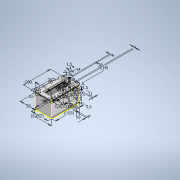
# Autodesk Inventor part: Box-Bildschirm.v2
Saved by Autodesk Inventor 2020 (Build 240168000, 168)
## iProperties
Created: 2019-08-23
Part Number: Box-Bildschirm.v2
Material: Generisch
Document SubType Name: Modeling
Designer: Admin
Density: 1 g/cm^3
Appearance: Vorgabe
Author: Admin
Autodesk Inventor part; units mm, degrees
ref_plane "YZ Plane" through (0, 0, 0) normal (1, 0, 0) x (0, 1, 0)
ref_plane "XZ Plane" through (0, 0, 0) normal (0, 1, 0) x (-1, 0, 0)
ref_plane "XY Plane" through (0, 0, 0) normal (0, 0, 1) x (1, 0, 0)
sketch "Skizze1" plane through (0, 0, 0) normal (0, 1, 0) x (-1, 0, 0)
  line L0 (0, 0) -> (56, 0)
  line L1 (56, 0) -> (56, 100)
  line L2 (56, 100) -> (0, 100)
  line L3 (0, 100) -> (0, 0)
  line L4 (57.5, 101.5) -> (-1.5, 101.5)
  line L5 (-1.5, 101.5) -> (-1.5, -1.5)
  line L6 (-1.5, -1.5) -> (57.5, -1.5)
  line L7 (57.5, -1.5) -> (57.5, 101.5)
  line L8 (42, 89) -> (14, 89)
  line L9 (14, 89) -> (14, 11)
  line L10 (14, 11) -> (42, 11)
  line L11 (42, 11) -> (42, 89)
  line L12 (38, 85) -> (18, 85)
  line L13 (18, 85) -> (18, 15)
  line L14 (18, 15) -> (38, 15)
  line L15 (38, 15) -> (38, 85)
  line L16 (56, 100) -> (56, 101.5)
  line L17 (56, 0) -> (56, -1.5)
  line L18 (0, -1.5) -> (0, 0)
  line L19 (0, 100) -> (0, 101.5)
  dimension "d0" = 100
  dimension "d1" = 56
  dimension "d2" = 1.5
  dimension "d3" = 1.5
  dimension "d4" = 1.5
  dimension "d5" = 1.5
  dimension "d6" = 28
  dimension "d7" = 78
  dimension "d8" = 11
  dimension "d9" = 11
  dimension "d10" = 4
  dimension "d11" = 4
  dimension "d12" = 4
  dimension "d13" = 4
  dimension "d14" = 14
  dimension "d15" = 14
  constraints: 40 end point, 8 parallel, 6 point on line, 5 perpendicular, 4 horizontal, 1 vertical
  measures "d0" distance between parallel lines of L2 L0
  measures "d1" distance between parallel lines of L3 L1
  measures "d2" distance between parallel lines of L4 L2
  measures "d3" distance from line of L6 L0.start
  measures "d4" distance between parallel lines of L5 L3
  measures "d5" distance between parallel lines of L1 L7
  measures "d6" distance between parallel lines of L9 L11
  measures "d7" distance between parallel lines of L8 L10
  measures "d8" distance between parallel lines of L0 L10
  measures "d9" distance between parallel lines of L2 L8
  measures "d10" distance between parallel lines of L14 L10
  measures "d11" distance between parallel lines of L8 L12
  measures "d12" distance between parallel lines of L15 L11
  measures "d13" distance between parallel lines of L13 L9
  measures "d14" distance between parallel lines of L1 L11
  measures "d15" distance between parallel lines of L3 L9
extrude "Extrusion1" add sketch "Skizze1" along normal blind 3 and the other way blind 55 contours L18 L6 L5 L4 L19 L3 | L0 L17 L6 L18 | L1 L16 L4 L7 L6 L17 | L19 L4 L16 L2
extrude "Extrusion2" add sketch "Skizze1" along normal blind 3 contours L3 L2 L1 L0
extrude "Extrusion3" add sketch "Skizze1" along normal blind 1.5 contours L11 L10 L9 L8
sketch "Skizze2" plane through (0, 0, 0) normal (0, -1, 0) x (1, 0, 0)
  line L0 (-9, 91) -> (-47, 91)
  line L1 (-47, 91) -> (-47, 9)
  line L2 (-47, 9) -> (-9, 9)
  line L3 (-9, 9) -> (-9, 91)
  line L4 (0, 0) -> (-56, 0) projected
  line L5 (-56, 0) -> (-56, 100) projected
  line L6 (-7.5, 92.5) -> (-48.5, 92.5)
  line L7 (-48.5, 92.5) -> (-48.5, 7.5)
  line L8 (-48.5, 7.5) -> (-7.5, 7.5)
  line L9 (-7.5, 7.5) -> (-7.5, 92.5)
  line L10 (-47, 91) -> (-41, 91)
  line L11 (-47, 85) -> (-47, 91)
  line L12 (-9, 91) -> (-15, 91)
  line L13 (-9, 85) -> (-9, 91)
  line L14 (-9, 9) -> (-15, 9)
  line L15 (-9, 15) -> (-9, 9)
  line L16 (-47, 9) -> (-41, 9)
  line L17 (-47, 15) -> (-47, 9)
  line L18 (-38, 85) -> (-38, 15) projected
  line L19 (-18, 15) -> (-18, 85) projected
  line L20 (-15, 86) -> (-41, 86)
  line L21 (-41, 86) -> (-41, 14)
  line L22 (-41, 14) -> (-15, 14)
  line L23 (-15, 14) -> (-15, 86)
  line L24 (-14, 11) -> (-14, 89) projected
  line L25 (-13.5, 87.5) -> (-42.5, 87.5)
  line L26 (-42.5, 87.5) -> (-42.5, 12.5)
  line L27 (-42.5, 12.5) -> (-13.5, 12.5)
  line L28 (-13.5, 12.5) -> (-13.5, 87.5)
  dimension "d26" = 82
  dimension "d27" = 38
  dimension "d28" = 9
  dimension "d29" = 9
  dimension "d30" = 1.5
  dimension "d31" = 1.5
  dimension "d32" = 1.5
  dimension "d33" = 1.5
  dimension "d39" = 6
  dimension "d40" = 20
  dimension "d41" = 26
  dimension "d42" = 72
  dimension "d43" = 6
  dimension "d44" = 5
  dimension "d45" = 1
  dimension "d46" = 1.5
  dimension "d47" = 1.5
  dimension "d48" = 1.5
  dimension "d49" = 1.5
  constraints: 48 end point, 8 horizontal, 8 parallel, 4 perpendicular
  measures "d26" distance between parallel lines of L0 L2
  measures "d27" distance between parallel lines of L1 L3
  measures "d28" distance between parallel lines of L4 L2
  measures "d29" distance between parallel lines of L5 L1
  measures "d30" distance between parallel lines of L6 L0
  measures "d31" distance between parallel lines of L7 L1
  measures "d32" distance between parallel lines of L3 L9
  measures "d33" distance between parallel lines of L8 L2
  measures "d39" distance from line of L3 L14.end
  measures "d40" distance between parallel lines of L18 L19
  measures "d41" distance between parallel lines of L21 L23
  measures "d42" distance between parallel lines of L22 L20
  measures "d43" distance between parallel lines of L1 L21
  measures "d44" distance between parallel lines of L0 L20
  measures "d45" distance between parallel lines of L24 L23
  measures "d46" distance between parallel lines of L25 L20
  measures "d47" distance between parallel lines of L22 L27
  measures "d48" distance between parallel lines of L28 L23
  measures "d49" distance between parallel lines of L26 L21
extrude "Extrusion4" add sketch "Skizze2" along normal blind 2.5 contours L27 L26 L25 L24 | L24 L25 L28 L27
sketch "Skizze3" plane through (0, 0, 0) normal (0, -1, 0) x (1, 0, 0)
  line L0 (-8, 91) -> (-46, 91)
  line L1 (-46, 91) -> (-46, 9)
  line L2 (-46, 9) -> (-8, 9)
  line L3 (-8, 9) -> (-8, 91)
  line L4 (-56, 100) -> (0, 100) projected
  line L5 (-56, 0) -> (-56, 100) projected
  line L6 (-6.5, 92.5) -> (-47.5, 92.5)
  line L7 (-47.5, 92.5) -> (-47.5, 7.5)
  line L8 (-47.5, 7.5) -> (-6.5, 7.5)
  line L9 (-6.5, 7.5) -> (-6.5, 92.5)
  arc A0 (-14, 91) -> (-8, 85) centre (-8, 91) ccw
  arc A1 (-8, 15) -> (-14, 9) centre (-8, 9) ccw
  arc A2 (-46, 85) -> (-40, 91) centre (-46, 91) ccw
  arc A3 (-40, 9) -> (-46, 15) centre (-46, 9) ccw
  line L10 (-6.5, 92.5) -> (0, 92.5)
  line L11 (0, 92.5) -> (0, 88.5)
  line L12 (0, 88.5) -> (-6.5, 88.5)
  line L13 (-6.5, 88.5) -> (-6.5, 92.5)
  line L14 (0, 100) -> (0, 0) projected
  line L15 (-47.5, 88.5) -> (-56, 88.5)
  line L16 (-56, 88.5) -> (-56, 92.5)
  line L17 (-56, 92.5) -> (-47.5, 92.5)
  line L18 (-47.5, 92.5) -> (-47.5, 88.5)
  line L19 (-6.5, 26.5) -> (0, 26.5)
  line L20 (0, 26.5) -> (0, 22.5)
  line L21 (0, 22.5) -> (-6.5, 22.5)
  line L22 (-6.5, 22.5) -> (-6.5, 26.5)
  line L23 (-47.5, 26.5) -> (-56, 26.5)
  line L24 (-56, 26.5) -> (-56, 22.5)
  line L25 (-56, 22.5) -> (-47.5, 22.5)
  line L26 (-47.5, 22.5) -> (-47.5, 26.5)
  point P0 (0, 26.5)
  point P1 (-6.5, 88.5)
  dimension "d52" = 38
  dimension "d53" = 82
  dimension "d54" = 9
  dimension "d55" = 10
  dimension "d56" = 1.5
  dimension "d57" = 1.5
  dimension "d58" = 1.5
  dimension "d59" = 1.5
  dimension "d60" = 6
  dimension "d101" = 6.5
  dimension "d102" = 4
  dimension "d103" = 0
  dimension "d104" = 6.5
  dimension "d105" = 4
  dimension "d106" = 70
  dimension "d107" = 0
  dimension "d108" = 4
  dimension "d109" = 70
  dimension "d110" = 66
  constraints: 48 end point, 15 point on line, 12 parallel, 8 point on circle, 6 horizontal, 6 perpendicular, 4 centre point, 4 coincident
  measures "d52" distance between parallel lines of L1 L3
  measures "d53" distance between parallel lines of L0 L2
  measures "d54" distance between parallel lines of L4 L0
  measures "d55" distance between parallel lines of L5 L1
  measures "d56" distance between parallel lines of L9 L3
  measures "d57" distance between parallel lines of L1 L7
  measures "d58" distance between parallel lines of L0 L6
  measures "d59" distance between parallel lines of L2 L8
  measures "d60" distance of L0.start A0.start
  measures "d101" distance between parallel lines of L9 L11
  measures "d102" distance between parallel lines of L10 L12
  measures "d103" distance from line of L6.start L10
  measures "d104" distance between parallel lines of L14 L9
  measures "d105" distance between parallel lines of L19 L21
  measures "d106" distance between parallel lines of L21 L10
  measures "d107" distance from line of L6.end L17
  measures "d108" distance between parallel lines of L17 L15
  measures "d109" distance between parallel lines of L25 L17
  measures "d110" distance between parallel lines of L23 L17
extrude "Extrusion5" add sketch "Skizze3" along normal blind 8 contours A2 L1 L0
extrude "Extrusion6" add sketch "Skizze3" along normal blind 8 contours L3 A0 L0
extrude "Extrusion7" add sketch "Skizze3" along normal blind 8 contours L3 L2 A1
extrude "Extrusion8" add sketch "Skizze3" along normal blind 8 contours A3 L2 L1
extrude "Extrusion9" add sketch "Skizze3" along normal blind 10 contours L6 L9 L8 L7
sketch "Skizze4" plane through (1.5, 3, -1.5) normal (0, 0, -1) x (-1, 0, 0)
  line L0 (36, -48) -> (39, -48)
  line L1 (39, -48) -> (39, -36)
  line L2 (39, -36) -> (36, -36)
  line L3 (36, -36) -> (36, -48)
  line L4 (59, -58) -> (0, -58) projected
  line L5 (1.5, -3) -> (57.5, -3) projected
  line L6 (59, -58) -> (59, 0) projected
  line L7 (0, -58) -> (0, 0) projected
  line L8 (34.5, -49.5) -> (40.5, -49.5)
  line L9 (40.5, -49.5) -> (40.5, -34.5)
  line L10 (40.5, -34.5) -> (34.5, -34.5)
  line L11 (34.5, -34.5) -> (34.5, -49.5)
  line L12 (34.5, -48) -> (31.5, -48)
  line L13 (31.5, -48) -> (31.5, -36)
  line L14 (31.5, -36) -> (34.5, -36)
  line L15 (34.5, -36) -> (34.5, -48)
  line L16 (34.5, -49.5) -> (30, -49.5)
  line L17 (30, -49.5) -> (30, -34.5)
  line L18 (30, -34.5) -> (34.5, -34.5)
  line L19 (34.5, -34.5) -> (34.5, -49.5)
  circle A0 centre (10, -43.4234) radius 1.75
  line L20 (6.75, -46.6734) -> (13.25, -46.6734)
  line L21 (13.25, -46.6734) -> (13.25, -40.1734)
  line L22 (13.25, -40.1734) -> (6.75, -40.1734)
  line L23 (6.75, -40.1734) -> (6.75, -46.6734)
  line L24 (5.25, -48.1734) -> (14.75, -48.1734)
  line L25 (14.75, -48.1734) -> (14.75, -38.6734)
  line L26 (14.75, -38.6734) -> (5.25, -38.6734)
  line L27 (5.25, -38.6734) -> (5.25, -48.1734)
  point P0 (34.5, -34.5)
  dimension "d71" = 3
  dimension "d72" = 12
  dimension "d73" = 55
  dimension "d74" = 10
  dimension "d75" = 59
  dimension "d76" = 36
  dimension "d77" = 20
  dimension "d119" = 1.5
  dimension "d120" = 1.5
  dimension "d121" = 1.5
  dimension "d122" = 1.5
  dimension "d123" = 3
  dimension "d124" = 1.5
  dimension "d125" = 12
  dimension "d126" = 1.5
  dimension "d127" = 3.5
  dimension "d128" = 10
  dimension "d129" = 6.5
  dimension "d130" = 6.5
  dimension "d131" = 3.25
  dimension "d132" = 3.25
  dimension "d133" = 1.5
  dimension "d134" = 1.5
  dimension "d135" = 1.5
  dimension "d136" = 1.5
  constraints: 48 end point, 12 parallel, 6 horizontal, 6 perpendicular, 1 centre point, 1 point on line
  measures "d71" distance between parallel lines of L1 L3
  measures "d72" distance between parallel lines of L2 L0
  measures "d73" distance between parallel lines of L4 L5
  measures "d74" distance between parallel lines of L4 L0
  measures "d75" distance between parallel lines of L6 L7
  measures "d76" distance between parallel lines of L7 L3
  measures "d77" distance between parallel lines of L6 L1
  measures "d119" distance between parallel lines of L3 L11
  measures "d120" distance between parallel lines of L9 L1
  measures "d121" distance between parallel lines of L10 L2
  measures "d122" distance between parallel lines of L0 L8
  measures "d123" distance between parallel lines of L19 L13
  measures "d124" distance between parallel lines of L13 L17
  measures "d125" distance between parallel lines of L12 L14
  measures "d126" distance between parallel lines of L12 L16
  measures "d127" diameter of A0
  measures "d128" distance from line of L7 A0.centre
  measures "d129" distance between parallel lines of L21 L23
  measures "d130" distance between parallel lines of L20 L22
  measures "d131" distance from line of L20 A0.centre
  measures "d132" distance from line of L23 A0.centre
  measures "d133" distance between parallel lines of L27 L23
  measures "d134" distance between parallel lines of L25 L21
  measures "d135" distance between parallel lines of L26 L22
  measures "d136" distance between parallel lines of L24 L20
extrude "Extrusion10" cut sketch "Skizze4" against normal blind 1.5 contours L3 L2 L1 L0 | L12 L13 L14 L11
sketch "Skizze5" plane through (1.5, -55, -1.5) normal (1, 0, 0) x (0, 0, -1)
  line L0 (0, 0) -> (-103, 0)
  line L1 (-103, 0) -> (-103, 1.5)
  line L2 (-103, 1.5) -> (0, 1.5)
  line L3 (0, 1.5) -> (0, 0)
  line L4 (0, 0) -> (0, 58) projected
  line L5 (-103, 0) -> (-103, 58) projected
  point P0 (-1.5, 55)
  dimension "d80" = 1.5
  dimension "d81" = 103
  dimension "d82" = 103
  constraints: 8 end point, 2 parallel, 1 horizontal, 1 perpendicular
  measures "d80" distance between parallel lines of L0 L2
  measures "d81" distance between parallel lines of L4 L5
  measures "d82" distance between parallel lines of L1 L3
extrude "Extrusion11" add sketch "Skizze5" along normal blind 1.5
sketch "Skizze6" plane through (-57.5, -55, 101.5) normal (-1, 0, 0) x (0, 0, 1)
  line L0 (0, 0) -> (-101.5, 0)
  line L1 (-101.5, 0) -> (-101.5, 1.5)
  line L2 (-101.5, 1.5) -> (0, 1.5)
  line L3 (0, 1.5) -> (0, 0)
  line L4 (-101.5, 1.5) -> (-121.5, 1.5)
  line L5 (-121.5, 1.5) -> (-121.5, 31.5)
  line L6 (-121.5, 31.5) -> (-101.5, 31.5)
  line L7 (-101.5, 31.5) -> (-101.5, 1.5)
  line L8 (-101.5, 0) -> (-101.5, 55) projected
  arc A0 (-121.5, 31.5) -> (-121.5, 1.5) centre (-121.5, 16.5) ccw
  circle A1 centre (-121.5, 16.5) radius 10
  dimension "d85" = 1.5
  dimension "d86" = 101.5
  dimension "d90" = 30
  dimension "d91" = 20
  dimension "d96" = 20
  constraints: 16 end point, 4 perpendicular, 2 centre point, 2 horizontal, 2 parallel, 2 point on circle, 2 tangent, 1 coincident
  measures "d85" distance between parallel lines of L2 L0
  measures "d86" distance between parallel lines of L1 L3
  measures "d90" distance between parallel lines of L6 L4
  measures "d91" diameter of A1
  measures "d96" distance between parallel lines of L7 L5
extrude "Extrusion12" add sketch "Skizze6" along normal blind 1.5 contours L0 L1 L2 L3
extrude "Extrusion13" cut sketch "Skizze6" against normal blind 2.5 contours L4 L5 A1 L6 L7 | A0 L5 A1
extrude "Extrusion14" add sketch "Skizze6" against normal blind 2.5 contours L4 L5 A1 L6 L7 | A0 L5 A1
sketch "Skizze7" plane through (0, -55, 0) normal (0, -1, 0) x (1, 0, 0)
  line L0 (-57.5, -1.5) -> (3, -1.5) projected
  line L1 (-59, 101.5) -> (3, 101.5) projected
  line L2 (-59, 0) -> (-59, 101.5) projected
  line L3 (3, 101.5) -> (3, -1.5) projected
  point P0 (0, 0)
  dimension "d97" = 103
  dimension "d98" = 62
  measures "d97" distance between parallel lines of L0 L1
  measures "d98" distance between parallel lines of L2 L3
sketch "Skizze8" plane through (-57.5, 3, 101.5) normal (0, 0, 1) x (1, 0, 0)
  line L0 (0, 0) -> (0, -56.5) projected
  line L1 (59, -56.5) -> (59, 0) projected
  line L2 (-1.5, -58) -> (-1.5, -56.5) projected
  line L3 (60.5, -56.5) -> (60.5, -58) projected
  point P0 (57.5, -3)
  dimension "d99" = 59
  dimension "d100" = 62
  measures "d99" distance between parallel lines of L0 L1
  measures "d100" distance between parallel lines of L2 L3
extrude "Extrusion15" add sketch "Skizze3" along normal blind 25 contours L23 L7 L25 L5
extrude "Extrusion16" add sketch "Skizze3" along normal blind 25 contours L17 L7 L15 L5
extrude "Extrusion17" add sketch "Skizze3" along normal blind 25 contours L14 L21 L9 L19
extrude "Extrusion18" add sketch "Skizze3" along normal blind 25 contours L11 L12 L9 L10
extrude "Extrusion19" add sketch "Skizze4" along normal blind 5 and the other way blind 6.5 contours L11 L10 L9 L8 | L16 L17 L18 L11 L14 L13 L12
extrude "Extrusion20" cut sketch "Skizze4" against normal blind 1.5 contours A0
extrude "Extrusion21" add sketch "Skizze4" against normal blind 3.5 contours L27 L26 L25 L24
